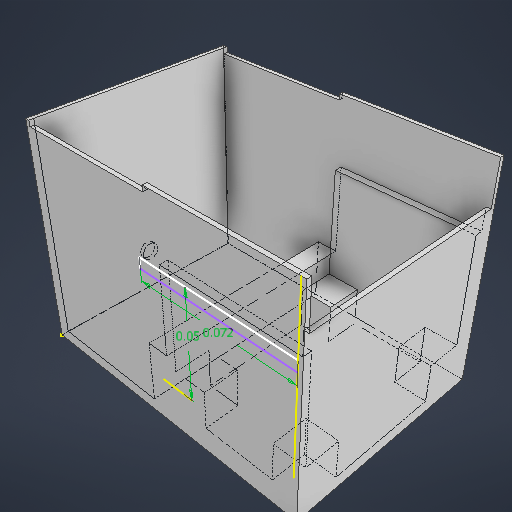
# Autodesk Inventor part: FINALE
Saved by Autodesk Inventor 2026.1 (Build 301233020, 233B)
## iProperties
Created: 2026-03-16
Part Number: FINALE
Material: Generic
Document SubType Name: Modeling
Designer: ktjau
Density: 1 g/cm^3
Appearance: Default
Author: ktjau
Autodesk Inventor part; units mm, degrees
ref_plane "YZ Plane" through (0, 0, 0) normal (1, 0, 0) x (0, 1, 0)
ref_plane "XZ Plane" through (0, 0, 0) normal (0, 1, 0) x (-1, 0, 0)
ref_plane "XY Plane" through (0, 0, 0) normal (0, 0, 1) x (1, 0, 0)
sketch "Sketch1" plane through (0, 0, 0) normal (0, 1, 0) x (-1, 0, 0)
  line L0 (0, 0) -> (-134, 0)
  line L1 (-134, 0) -> (-134, -96)
  line L2 (-134, -96) -> (0, -96)
  line L3 (0, -96) -> (0, 0)
  line L4 (0, 0) -> (-2, 0)
  line L5 (-2, 0) -> (-2, -2)
  line L6 (-2, -2) -> (0, -2)
  line L7 (0, -2) -> (0, 0)
  line L8 (-134, -96) -> (-132, -96)
  line L9 (-132, -96) -> (-132, -94)
  line L10 (-132, -94) -> (-134, -94)
  line L11 (-134, -94) -> (-134, -96)
  line L12 (-2, -2) -> (-132, -2)
  line L13 (-132, -2) -> (-132, -94)
  line L14 (-132, -94) -> (-2, -94)
  line L15 (-2, -94) -> (-2, -2)
  line L16 (-132, -94) -> (-68, -94)
  line L17 (-68, -94) -> (-68, -74)
  line L18 (-68, -74) -> (-132, -74)
  line L19 (-132, -74) -> (-132, -94)
  line L20 (-132, -2) -> (-68, -2)
  line L21 (-68, -2) -> (-68, -22)
  line L22 (-68, -22) -> (-132, -22)
  line L23 (-132, -22) -> (-132, -2)
  line L24 (-132, -74) -> (-71.6783, -74)
  line L25 (-71.6783, -22) -> (-132, -22)
  line L26 (-71.6783, -74) -> (-71.6783, -22)
  line L27 (-71.6783, -88.5049) -> (-132, -88.5049)
  line L28 (-132, -88.5049) -> (-132, -7.5049)
  line L29 (-132, -7.5049) -> (-71.6783, -7.5049)
  line L30 (-71.6783, -7.5049) -> (-71.6783, -88.5049)
  line L31 (-68, -94) -> (-58.2781, -94)
  line L32 (-58.2781, -94) -> (-58.2781, -2)
  line L33 (-58.2781, -2) -> (-68, -2)
  line L34 (-68, -2) -> (-68, -94)
  line L35 (-2, -94) -> (-58.2781, -94)
  line L36 (-58.2781, -94) -> (-58.2781, -2)
  line L37 (-58.2781, -2) -> (-2, -2)
  line L38 (-2, -2) -> (-2, -94)
  line L39 (-68, -74) -> (-83.3567, -74)
  line L40 (-83.3567, -74) -> (-83.3567, -94)
  line L41 (-83.3567, -94) -> (-68, -94)
  line L42 (-68, -94) -> (-68, -74)
  line L43 (-132, -74) -> (-117.3588, -74)
  line L44 (-117.3588, -74) -> (-117.3588, -94)
  line L45 (-117.3588, -94) -> (-132, -94)
  line L46 (-132, -94) -> (-132, -74)
  line L47 (-68, -22) -> (-83.3567, -22)
  line L48 (-83.3567, -22) -> (-83.3567, -2)
  line L49 (-83.3567, -2) -> (-68, -2)
  line L50 (-68, -2) -> (-68, -22)
  line L51 (-117.3588, -22) -> (-132, -22)
  line L52 (-132, -22) -> (-132, -2)
  line L53 (-132, -2) -> (-117.3588, -2)
  line L54 (-117.3588, -2) -> (-117.3588, -22)
  line L55 (-68, -5.7143) -> (-132, -5.7143)
  line L56 (-132, -5.7143) -> (-132, -2)
  line L57 (-132, -2) -> (-68, -2)
  line L58 (-68, -2) -> (-68, -5.7143)
  line L59 (-68, -94) -> (-132, -94)
  line L60 (-132, -94) -> (-132, -90.4872)
  line L61 (-132, -90.4872) -> (-68, -90.4872)
  line L62 (-68, -90.4872) -> (-68, -94)
  line L63 (-132, -92.2436) -> (-29, -92.2436)
  line L64 (-29, -92.2436) -> (-29, -2.2436)
  line L65 (-29, -2.2436) -> (-132, -2.2436)
  line L66 (-132, -2.2436) -> (-132, -92.2436)
  point P0 (-83.3567, -2)
  point P1 (-83.3567, -7.5049)
  point P2 (-117.3588, -7.5049)
  point P3 (-132, -7.5049)
  point P4 (-132, -88.5049)
  point P5 (-117.3588, -88.5049)
  point P6 (-83.3567, -88.5049)
  dimension "d0" = 134
  dimension "d1" = 96
  dimension "d2" = 2
  dimension "d3" = 2
  dimension "d4" = 2
  dimension "d5" = 2
  dimension "d6" = 64
  dimension "d7" = 64
  dimension "d9" = 20
  dimension "d10" = 20
  dimension "d11" = 81
  dimension "d22" = 5.5049
  dimension "d23" = 90
  dimension "d24" = 103
  constraints: 134 end point, 32 parallel, 17 perpendicular, 16 horizontal, 12 point on line, 1 collinear, 1 midpoint
  measures "d0" distance of L1.end L2.end
  measures "d1" distance of L0.end L1.end
  measures "d2" distance of L5.end L6.end
  measures "d3" distance of L4.end L5.end
  measures "d4" distance of L8.end L9.end
  measures "d5" distance of L9.end L10.end
  measures "d6" distance of L17.end L18.end
  measures "d7" distance of L21.end L22.end
  measures "d9" distance of L16.end L17.end
  measures "d10" distance of L20.end L21.end
  measures "d11" distance of L29.end L27.start
  measures "d22" distance between parallel lines of L20 L29
  measures "d23" distance between parallel lines of L65 L63
  measures "d24" distance between parallel lines of L66 L64
extrude "Extrusion1" add sketch "Sketch1" along normal blind 100 contours L3 L6 L5 L0 | L5 L12 L13 L10 L1 L0 | L3 L2 L9 L14 L15 L6 | L10 L9 L2 L1
extrude "Extrusion2" add sketch "Sketch1" along normal blind 20 contours L13 L63 L44 L14 | L21 L65 L48 L12 | L13 L61 L44 L63 | L21 L55 L48 L65 | L14 L40 L63 L17 | L13 L27 L44 L61 | L54 L65 L13 L12 | L21 L22 L30 L29 L48 L55 | L63 L40 L61 L17 | L13 L18 L44 L27 | L54 L55 L13 L65 | L61 L40 L27 L30 L18 L17 | L54 L29 L13 L55 | L29 L30 L22 L48 | L13 L29 L54 L22 | L40 L18 L30 L27
extrude "Extrusion3" add sketch "Sketch1" along normal blind 30 contours L32 L65 L21 L12 | L32 L63 L17 L34 L21 L65 | L14 L17 L63 L32
extrude "Extrusion4" add sketch "Sketch1" along normal blind 2 contours L15 L14 L32 L63 L64 L65 L12 | L65 L64 L63 L32 | L44 L63 L40 L14 | L48 L65 L54 L12 | L44 L61 L40 L63 | L48 L55 L54 L65 | L13 L18 L44 L27 | L44 L27 L40 L61 | L48 L29 L54 L55 | L34 L18 L26 L22 | L13 L22 L26 L18 | L44 L18 L40 L27 | L48 L22 L54 L29 | L29 L30 L22 L48 | L13 L29 L54 L22 | L40 L18 L30 L27
sketch "Sketch2" plane through (0, 0, 0) normal (0, 0, 1) x (1, 0, 0)
  line L0 (132, 20) -> (132, 100) projected
  line L1 (132, 70) -> (60, 70)
  line L2 (83.3567, 20) -> (68, 20) projected
  line L3 (60, 70) -> (132, 70)
  line L4 (132, 70) -> (132, 65.2658)
  line L5 (132, 65.2658) -> (60, 65.2658)
  line L6 (60, 65.2658) -> (60, 70)
  point P0 (0, 0)
  dimension "d20" = 50
  dimension "d21" = 72
  constraints: 10 end point, 2 horizontal, 2 parallel, 2 point on line, 1 perpendicular
  measures "d20" distance between parallel lines of L1 L2
  measures "d21" distance of L1.start L1.end
extrude "Extrusion5" add sketch "Sketch1" along normal blind 70 contours L13 L63 L44 L14 | L21 L65 L48 L12 | L13 L61 L44 L63 | L44 L63 L40 L14 | L48 L65 L54 L12 | L21 L55 L48 L65 | L14 L40 L63 L17 | L44 L61 L40 L63 | L54 L65 L13 L12 | L48 L55 L54 L65 | L63 L40 L61 L17 | L54 L55 L13 L65
sketch "Sketch3" plane through (0, 100, 0) normal (0, 1, 0) x (1, 0, 0)
  line L0 (0, 0) -> (134, 0) projected
  line L1 (2.0076, 96.0653) -> (65.0076, 96.0653)
  line L2 (65.0076, 96.0653) -> (65.0076, 0)
  line L3 (65.0076, 0) -> (2.0076, 0)
  line L4 (2.0076, 0) -> (2.0076, 96.0653)
  dimension "d27" = 63
  constraints: 8 end point, 2 parallel, 1 horizontal, 1 perpendicular, 1 point on line
  measures "d27" distance between parallel lines of L2 L4
extrude "Extrusion6" cut sketch "Sketch3" against normal blind 2.5
sketch "Sketch4" plane through (0, 0, -96) normal (-1, 0, 0) x (0, 0, 1)
  line L0 (2, 2) -> (2, 100) projected
  line L1 (94, 2) -> (2, 2) projected
  line L2 (2, 2) -> (94, 2)
  circle A0 centre (48, 20.0516) radius 4
  point P0 (96, 0)
  dimension "d30" = 8
  constraints: 2 end point, 1 centre point, 1 collinear
  measures "d30" diameter of A0
sketch "Sketch5" plane through (0, 100, 0) normal (0, 1, 0) x (1, 0, 0)
  line L0 (134, 0) -> (134, 96) projected
  line L1 (132, 94) -> (134, 94)
  line L2 (134, 94) -> (134, 2)
  line L3 (134, 2) -> (132, 2)
  line L4 (132, 2) -> (132, 94)
  point P0 (0, 0)
  dimension "d31" = 92
  constraints: 8 end point, 2 parallel, 1 horizontal, 1 perpendicular, 1 point on line
  measures "d31" distance from line of L3 L1.start
extrude "Extrusion7" cut sketch "Sketch5" against normal blind 20
extrude "Extrusion8" cut sketch "Sketch4" against normal blind 20
body "Solid1"
